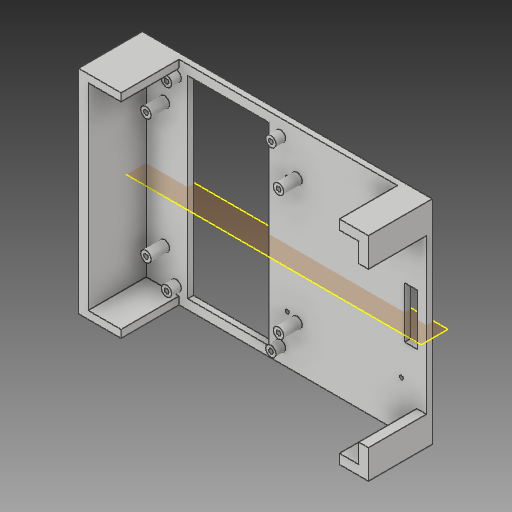
# Autodesk Inventor part: Case
Saved by Autodesk Inventor 2019 (Build 230136000, 136)
## iProperties
Created: 2019-03-10
Part Number: Case
Material: Generic
Document SubType Name: Modeling
Designer: savo
Density: 1 g/cm^3
Appearance: Default
Author: savo
Autodesk Inventor part; units mm, degrees
ref_plane "YZ Plane" through (0, 0, 0) normal (1, 0, 0) x (0, 1, 0)
ref_plane "XZ Plane" through (0, 0, 0) normal (0, 1, 0) x (-1, 0, 0)
ref_plane "XY Plane" through (0, 0, 0) normal (0, 0, 1) x (1, 0, 0)
sketch "Sketch1" plane through (0, 0, 0) normal (0, 0, 1) x (1, 0, 0)
  line L0 (8, 55) -> (-142, 55)
  line L1 (-142, 55) -> (-142, -55)
  line L2 (-142, -55) -> (8, -55)
  line L3 (8, -55) -> (8, 55)
  line L4 (8, 0) -> (-142, 0) construction
  line L5 (-114.5, 49) -> (-74.5, 49) projected
  line L6 (-74.5, 49) -> (-74.5, -49) projected
  line L7 (-74.5, -49) -> (-114.5, -49) projected
  line L8 (-114.5, -49) -> (-114.5, 49) projected
  line L9 (-115.5, 50) -> (-73.5, 50)
  line L10 (-73.5, 50) -> (-73.5, -50)
  line L11 (-73.5, -50) -> (-115.5, -50)
  line L12 (-115.5, -50) -> (-115.5, 50)
  line L13 (2.5, 12.5) -> (-2.5, 12.5) projected
  line L14 (-2.5, 12.5) -> (-2.5, -12.5) projected
  line L15 (-2.5, -12.5) -> (2.5, -12.5) projected
  line L16 (2.5, -12.5) -> (2.5, 12.5) projected
  line L17 (3.25, -13.25) -> (-3.25, -13.25)
  line L18 (-3.25, -13.25) -> (-3.25, 13.25)
  line L19 (-3.25, 13.25) -> (3.25, 13.25)
  line L20 (3.25, 13.25) -> (3.25, -13.25)
  point P0 (0, 0)
  dimension "d0" = 110
  dimension "d1" = 150
  dimension "d2" = 8
  dimension "d3" = 1
  dimension "d4" = 0.75
  constraints: 26 end point, 2 midpoint, 2 parallel, 1 horizontal, 1 perpendicular, 1 point on line, 6 other
  measures "d0" distance of L0.end L1.end
  measures "d1" distance of L0.start L0.end
  measures "d2" distance from line of L3 point (0, 0)
  measures "d3" distance between parallel lines of L8 L12
  measures "d4" distance between parallel lines of L15 L17
extrude "Extrusion1" add sketch "Sketch1" along normal blind 3 contours L3 L2 L1 L0
sketch "Sketch2" plane through (0, 0, 3) normal (0, 0, 1) x (1, 0, 0)
  circle A0 centre (-67.5, -47) radius 1.7 construction
  circle A1 centre (-67.5, 47) radius 1.7 construction
  circle A2 centre (-121.5, 47) radius 1.7 construction
  circle A3 centre (-121.5, -47) radius 1.7 construction
  line L0 (-64.5, 50) -> (-124.5, 50) construction
  line L1 (-124.5, 50) -> (-124.5, -50) construction
  line L2 (-124.5, -50) -> (-64.5, -50) construction
  line L3 (-64.5, -50) -> (-64.5, 50) construction
  circle A4 centre (-67.5, 47) radius 2.7
  circle A5 centre (-121.5, 47) radius 2.7
  circle A6 centre (-67.5, -47) radius 2.7
  circle A7 centre (-121.5, -47) radius 2.7
  point P0 (0, 0)
  dimension "d7" = 1
  constraints: 4 centre point, 3 equal radius
  measures "d7" radial gap between concentric circles of A1 A4
ref_plane "Work Plane1" through (-126.5, -50, 8) normal (0, 0, -1) x (0, 1, 0)
extrude "Extrusion2" add sketch "Sketch2" along normal up to surface (5 mm away)
sketch "Sketch3" plane through (-121.5, 47, 8) normal (0, 0, 1) x (1, 0, 0)
  circle A0 centre (54, -94) radius 1.7 construction
  circle A1 centre (54, 0) radius 1.7 construction
  circle A2 centre (0, 0) radius 1.7 construction
  circle A3 centre (0, -94) radius 1.7 construction
  line L0 (57, 3) -> (-3, 3) construction
  line L1 (-3, 3) -> (-3, -97) construction
  line L2 (-3, -97) -> (57, -97) construction
  line L3 (57, -97) -> (57, 3) construction
  circle A4 centre (0, 0) radius 2.7 construction
  point P0 (121.5, -47)
  constraints: 4 coincident
hole "Hole1" at (-121.5, 47, 8) at (-121.5, -47, 8) at (-67.5, -47, 8) at (-67.5, 47, 8) direction (0, 0, -1) diameter 2.459 depth 5 tip angle 118 thread size "M3x0.5" class "6H" standard "ANSI Metric M Profile"
sketch "Sketch4" plane through (0, 0, 0) normal (0, 0, -1) x (-1, 0, 0)
  circle A0 centre (64, -30) radius 1.2 construction
  circle A1 centre (64, 30) radius 1.2 construction
  circle A2 centre (5, 30) radius 1.2 construction
  circle A3 centre (5, -30) radius 1.2 construction
  line L0 (66.5, 32.5) -> (2.5, 32.5) construction
  line L1 (2.5, 32.5) -> (2.5, -32.5) construction
  line L2 (2.5, -32.5) -> (66.5, -32.5) construction
  line L3 (66.5, -32.5) -> (66.5, 32.5) construction
  point P0 (0, 0)
  constraints: 4 coincident
hole "Hole2" at (-5, -30, 0) at (-5, 30, 0) at (-64, 30, 0) at (-64, -30, 0) direction (0, 0, 1) diameter 2.013 end through all thread size "M2.5x0.45" class "6H" standard "ANSI Metric M Profile"
sketch "Sketch5" plane through (0, 0, 3) normal (0, 0, 1) x (1, 0, 0)
  circle A0 centre (-58.945, 32.258) radius 1.7 construction
  circle A1 centre (-127.525, -32.258) radius 1.7 construction
  circle A2 centre (-127.525, 32.258) radius 1.7 construction
  line L0 (-54.5, -35.56) -> (-54.5, 35.56) construction
  line L1 (-54.5, 35.56) -> (-131.97, 35.56) construction
  line L2 (-131.97, 35.56) -> (-131.97, -35.56) construction
  line L3 (-131.97, -35.56) -> (-54.5, -35.56) construction
  circle A3 centre (-127.525, 32.258) radius 2.7
  circle A4 centre (-58.945, 32.258) radius 2.7
  point P0 (0, 0)
  dimension "d24" = 1
  constraints: 2 centre point, 1 equal radius
  measures "d24" radial gap between concentric circles of A2 A3
ref_plane "Work Plane2" through (-134.4075, -35.56, 12.6) normal (0, 0, -1) x (0, 1, 0)
extrude "Extrusion3" add sketch "Sketch5" along normal up to surface (9.6 mm away)
sketch "Sketch6" plane through (-127.525, 32.258, 12.6) normal (0, 0, 1) x (1, 0, 0)
  circle A0 centre (0, 0) radius 2.7 projected
  circle A1 centre (68.58, 0) radius 2.7 projected
  point P0 (127.525, -32.258)
  constraints: 2 coincident
hole "Hole3" at (-127.525, 32.258, 12.6) at (-58.945, 32.258, 12.6) direction (0, 0, -1) diameter 2.459 depth 8.8 tip angle 118 thread size "M3x0.5" class "6H" standard "ANSI Metric M Profile"
ref_plane "Work Plane3" through (-142, 0, 0) normal (0, 1, 0) x (1, 0, 0)
mirror "Mirror1" about plane through (-142, 0, 0) normal (0, 1, 0) of "Extrusion3", "Hole3"
sketch "Sketch7" plane through (0, 0, 3) normal (0, 0, 1) x (1, 0, 0)
  circle A0 centre (-127.525, 32.258) radius 2.7 construction
  circle A1 centre (-58.945, 32.258) radius 2.7 construction
  circle A2 centre (-64, 30) radius 1.0065 construction
  circle A3 centre (-5, -30) radius 1.0065 construction
  circle A4 centre (-5, 30) radius 1.0065 construction
  circle A5 centre (-58.945, -32.258) radius 2.7 construction
  circle A6 centre (-64, -30) radius 1.0065 construction
  circle A7 centre (-67.5, -47) radius 2.7 construction
  circle A8 centre (-121.5, -47) radius 2.7 construction
  circle A9 centre (-121.5, 47) radius 2.7 construction
  circle A10 centre (-67.5, 47) radius 2.7 construction
  line L0 (-73.5, 50) -> (-73.5, -50) construction
  line L1 (-73.5, -50) -> (-115.5, -50) construction
  line L2 (-115.5, -50) -> (-115.5, 50) construction
  line L3 (-115.5, 50) -> (-73.5, 50) construction
  line L4 (-3.25, -13.25) -> (-3.25, 13.25) construction
  line L5 (-3.25, 13.25) -> (3.25, 13.25) construction
  line L6 (3.25, 13.25) -> (3.25, -13.25) construction
  line L7 (3.25, -13.25) -> (-3.25, -13.25) construction
  line L8 (8, 55) -> (-142, 55) construction
  line L9 (-142, 55) -> (-142, -55) construction
  line L10 (-142, -55) -> (8, -55) construction
  line L11 (8, -55) -> (8, 55) construction
  circle A11 centre (-127.525, -32.258) radius 2.7 construction
  line L12 (-142, 55) -> (-142, -55) projected
  line L13 (-142, -55) -> (8, -55) projected
  line L14 (-142, 55) -> (-137, 55)
  line L15 (-137, 55) -> (-137, -55)
  line L16 (-137, -55) -> (-142, -55)
  line L17 (-142, -55) -> (-142, 55)
  line L18 (8, 55) -> (-142, 55) projected
  line L19 (-120, 55) -> (-142, 55)
  line L20 (-142, 55) -> (-142, 51)
  line L21 (-142, 51) -> (-120, 51)
  line L22 (-120, 51) -> (-120, 55)
  line L23 (-142, 55) -> (-142, -55) projected
  line L24 (8, 0) -> (-142, 0)
  line L25 (8, -55) -> (-142, -55) construction
  line L26 (8, -55) -> (-142, -55)
  line L27 (-120, -51) -> (-120, -55)
  line L28 (8, 55) -> (-7, 55)
  line L29 (-7, 55) -> (-7, 50)
  line L30 (-7, 50) -> (8, 50)
  line L31 (8, 50) -> (8, 55)
  line L32 (8, -55) -> (-7, -55)
  line L33 (-7, -55) -> (-7, -50)
  line L34 (-7, -50) -> (8, -50)
  line L35 (8, -50) -> (8, -55)
  line L36 (-120, -51) -> (-142, -51)
  line L37 (-142, -51) -> (-142, -55)
  line L38 (-142, -55) -> (-120, -55)
  line L39 (-120, -55) -> (-120, -51)
  line L40 (8, 55) -> (3, 55)
  line L41 (3, 55) -> (3, 40)
  line L42 (3, 40) -> (8, 40)
  line L43 (8, 40) -> (8, 55)
  line L44 (8, -55) -> (8, 55) projected
  line L45 (8, -55) -> (3, -55)
  line L46 (3, -55) -> (3, -40)
  line L47 (3, -40) -> (8, -40)
  line L48 (8, -40) -> (8, -55)
  point P0 (0, 0)
  dimension "d34" = 5
  dimension "d35" = 22
  dimension "d36" = 4
  dimension "d37" = 15
  dimension "d38" = 5
  constraints: 64 end point, 14 parallel, 11 perpendicular, 7 horizontal, 6 point on line, 3 symmetric about line, 2 midpoint
  measures "d34" distance of L15.end L16.end
  measures "d35" distance of L21.end L20.end
  measures "d36" distance of L20.end L19.end
  measures "d37" distance of L41.end L40.end
  measures "d38" distance of L28.end L29.end
extrude "Extrusion4" add sketch "Sketch7" along normal blind 30 contours L14 L15 L21 L12 | L21 L15 L24 L12 | L18 L22 L21 L15 | L24 L15 L36 L12 | L36 L15 L13 L12 | L18 L41 L30 L29 | L36 L27 L13 L15 | L18 L31 L30 L41 | L44 L34 L46 L47 | L42 L41 L30 L43 | L35 L13 L46 L34 | L33 L34 L46 L13
body "Solid1"
